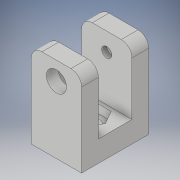
# Autodesk Inventor part: xTension
Saved by Autodesk Inventor 2019 (Build 230136000, 136)
## iProperties
Created: 2019-05-16
Part Number: xTension
Material: Generic
Document SubType Name: Modeling
Designer: Alex Jones
Density: 1 g/cm^3
Appearance: Default
Author: Alex Jones
Autodesk Inventor part; units mm, degrees
ref_plane "YZ Plane" through (0, 0, 0) normal (1, 0, 0) x (0, 1, 0)
ref_plane "XZ Plane" through (0, 0, 0) normal (0, 1, 0) x (-1, 0, 0)
ref_plane "XY Plane" through (0, 0, 0) normal (0, 0, 1) x (1, 0, 0)
sketch "Sketch1" plane through (0, 0, 0) normal (0, 1, 0) x (-1, 0, 0)
  line L0 (-7.5, 9) -> (7.5, 9)
  line L1 (7.5, 9) -> (7.5, -9)
  line L2 (7.5, -9) -> (-7.5, -9)
  line L3 (-7.5, -9) -> (-7.5, 9)
  line L4 (-7.5, 9) -> (7.5, -9) construction
  line L5 (7.5, 9) -> (-7.5, -9) construction
  point P0 (0, 0)
  dimension "d0" = 18
  dimension "d1" = 15
  constraints: 12 end point, 2 midpoint, 2 parallel, 1 horizontal, 1 perpendicular
  measures "d0" distance of L0.end L1.end
  measures "d1" distance of L1.end L2.end
extrude "Extrusion1" add sketch "Sketch1" along normal blind 25.4
sketch "Sketch2" plane through (0, 25.4, 0) normal (0, 1, 0) x (1, 0, 0)
  line L0 (12.4357, -5) -> (-12.4357, -5)
  line L1 (-12.4357, -5) -> (-12.4357, 5)
  line L2 (-12.4357, 5) -> (12.4357, 5)
  line L3 (12.4357, 5) -> (12.4357, -5)
  line L4 (12.4357, -5) -> (-12.4357, 5) construction
  line L5 (-12.4357, -5) -> (12.4357, 5) construction
  line L6 (7.5, 9) -> (-7.5, 9) projected
  point P0 (0, 0)
  dimension "d5" = 10
  constraints: 12 end point, 2 midpoint, 2 parallel, 1 horizontal, 1 perpendicular
  measures "d5" distance of L0.end L1.end
extrude "Extrusion2" cut sketch "Sketch2" against normal blind 19.05
sketch "Sketch3" plane through (7.5, 0, -9) normal (0, 0, -1) x (-1, 0, 0)
  line L0 (0, 25.4) -> (15, 25.4) projected
  line L1 (7.5, 25.4) -> (7.5, 0)
  circle A0 centre (7.5, 19.9547) radius 1.5
  dimension "d8" = 3
  constraints: 2 end point, 1 centre point, 1 midpoint, 1 point on line, 1 vertical
  measures "d8" diameter of A0
extrude "Extrusion3" cut sketch "Sketch3" against normal through all
fillet "Fillet1" radius 3.175 4 edges at (-7.5, 25.4, -7) (7.5, 25.4, -7) (-7.5, 25.4, 7) (7.5, 25.4, 7)
sketch "Sketch4" plane through (0, 0, 0) normal (0, -1, 0) x (1, 0, 0)
  circle A0 centre (0, 0) radius 2.75
  dimension "d12" = 5.5
  constraints: 1 centre point, 1 coincident
  measures "d12" diameter of A0
extrude "Extrusion4" cut sketch "Sketch4" against normal blind 19.05
sketch "Sketch5" plane through (0, 6.35, 0) normal (0, 1, 0) x (1, 0, 0)
  line L0 (-4.6188, 0) -> (-2.3094, 4)
  line L1 (-2.3094, 4) -> (2.3094, 4)
  line L2 (2.3094, 4) -> (4.6188, 0)
  line L3 (4.6188, 0) -> (2.3094, -4)
  line L4 (2.3094, -4) -> (-2.3094, -4)
  line L5 (-2.3094, -4) -> (-4.6188, 0)
  point P0 (0, 0)
  point P1 (0, 0)
  dimension "d15" = 8
  constraints: 12 end point, 1 coincident, 13 other
  measures "d15" distance between parallel lines of L4 L1
extrude "Extrusion5" cut sketch "Sketch5" against normal blind 2.54
sketch "Sketch6" plane through (-7.5, 0, 9) normal (0, 0, 1) x (1, 0, 0)
  circle A0 centre (7.5, 19.9547) radius 1.5 projected
  circle A1 centre (7.5, 19.9547) radius 3
  point P0 (7.5, 0)
  dimension "d18" = 6
  constraints: 1 centre point, 1 coincident
  measures "d18" diameter of A1
extrude "Extrusion6" cut sketch "Sketch6" against normal blind 2.5
sketch "Sketch7" plane through (7.5, 0, -9) normal (0, 0, -1) x (-1, 0, 0)
  circle A0 centre (7.5, 19.9547) radius 1.5 projected
  line L0 (10.6129, 19.0812) -> (8.3, 16.822)
  line L1 (8.3, 16.822) -> (5.1871, 17.6955)
  line L2 (5.1871, 17.6955) -> (4.3871, 20.8282)
  line L3 (4.3871, 20.8282) -> (6.7, 23.0873)
  line L4 (6.7, 23.0873) -> (9.8129, 22.2138)
  line L5 (9.8129, 22.2138) -> (10.6129, 19.0812)
  point P0 (7.5, 0)
  dimension "d21" = 5.6
  constraints: 12 end point, 1 coincident, 13 other
  measures "d21" distance between parallel lines of L5 L2
extrude "Extrusion7" cut sketch "Sketch7" against normal blind 2.5
sketch "Sketch8" plane through (7.5, 0, -9) normal (0, 0, -1) x (-1, 0, 0)
  line L0 (9.8129, 22.2138) -> (10.6129, 19.0812) projected
  line L1 (10.6129, 19.0812) -> (8.3, 16.822) projected
  line L2 (8.3, 16.822) -> (5.1871, 17.6955) projected
  line L3 (5.1871, 17.6955) -> (4.3871, 20.8282) projected
  line L4 (4.3871, 20.8282) -> (6.7, 23.0873) projected
  line L5 (6.7, 23.0873) -> (9.8129, 22.2138) projected
  arc A0 (3.175, 25.4) -> (0, 22.225) centre (3.175, 22.225) ccw projected
  line L6 (0, 0) -> (0, 22.225) projected
  line L7 (15, 0) -> (0, 0) projected
  line L8 (15, 0) -> (15, 22.225) projected
  arc A1 (15, 22.225) -> (11.825, 25.4) centre (11.825, 22.225) ccw projected
  line L9 (3.175, 25.4) -> (11.825, 25.4) projected
  point P0 (7.5, 0)
extrude "Extrusion8" add sketch "Sketch8" along normal blind 1
sketch "Sketch9" plane through (-7.5, 0, 9) normal (0, 0, 1) x (1, 0, 0)
  circle A0 centre (7.5, 19.9547) radius 3 projected
  arc A1 (15, 22.225) -> (11.825, 25.4) centre (11.825, 22.225) ccw projected
  line L0 (3.175, 25.4) -> (11.825, 25.4) projected
  arc A2 (3.175, 25.4) -> (0, 22.225) centre (3.175, 22.225) ccw projected
  line L1 (0, 0) -> (0, 22.225) projected
  line L2 (15, 0) -> (0, 0) projected
  line L3 (15, 0) -> (15, 22.225) projected
  point P0 (7.5, 0)
extrude "Extrusion9" add sketch "Sketch9" along normal blind 1
body "Solid1"
